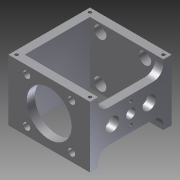
# Autodesk Inventor part: 13_0204_016
Saved by Autodesk Inventor 2012 SP1 (Build 160190100, 190)
## iProperties
Created: 2013-03-28
Part Number: 13_0204_016
Material: Default
Document SubType Name: Modeling
Designer: vogel
Density: 1 g/cm^3
Author: vogel
Autodesk Inventor part; units mm, degrees
note: some values were not read from the file. Chosen so that the rebuilt part matches the saved one: direction of "Bohrung2"; direction of "Bohrung3"; direction of "Bohrung4"; direction of "Bohrung5".
ref_plane "YZ Plane" through (0, 0, 0) normal (1, 0, 0) x (0, 1, 0)
ref_plane "XZ Plane" through (0, 0, 0) normal (0, 1, 0) x (-1, 0, 0)
sketch "Skizze1" plane through (0, 0, 0) normal (0, 0, 1) x (1, 0, 0)
  line L0 (-20, 20) -> (20, 20)
  line L1 (20, 20) -> (20, -20)
  line L2 (20, -20) -> (-20, -20)
  line L3 (-20, -20) -> (-20, 20)
  line L4 (-28, 0) -> (28, 0) projected
  line L5 (0, -28) -> (0, 28) projected
  line L6 (16, 16) -> (-16, 16)
  line L7 (-16, 16) -> (-16, -16)
  line L8 (-16, -16) -> (16, -16)
  line L9 (16, -16) -> (16, 16)
  point P0 (0, 0)
  dimension "d0" = 40
  dimension "d1" = 4
  constraints: 16 end point, 4 parallel, 3 perpendicular, 1 horizontal, 5 other
  measures "d0" distance of L2.end L0.start
  measures "d1" distance between parallel lines of L0 L6
extrude "Extrusion1" add sketch "Skizze1" along normal blind 30 contours L0 L5 L6 L7 L4 L3 | L0 L1 L4 L9 L6 L5 | L4 L7 L8 L5 L2 L3 | L1 L2 L5 L8 L9 L4
sketch "Skizze2" plane through (20, -20, 0) normal (1, 0, 0) x (0, 0, -1)
  line L0 (-30, 40) -> (-30, 0) projected
  line L1 (0, 0) -> (-30, 0) projected
  line L2 (0, 40) -> (-30, 40) projected
  line L3 (0, -8) -> (0, 48) projected
  line L4 (6, 20) -> (-36, 20) projected
  line L5 (-30, 36) -> (-28, 36)
  line L6 (-23, 31) -> (-23, 9)
  line L7 (-28, 4) -> (-30, 4)
  line L8 (-30, 4) -> (-30, 36)
  line L9 (0, 36) -> (-2, 36)
  line L10 (-7, 31) -> (-7, 9)
  line L11 (-2, 4) -> (0, 4)
  line L12 (0, 4) -> (0, 36)
  line L13 (-15, 40) -> (-15, 0)
  line L14 (0, 4) -> (-30, 4) projected
  arc A0 (-23, 31) -> (-28, 36) centre (-28, 31) ccw
  arc A1 (-28, 4) -> (-23, 9) centre (-28, 9) ccw
  arc A2 (-7, 9) -> (-2, 4) centre (-2, 9) ccw
  arc A3 (-2, 36) -> (-7, 31) centre (-2, 31) ccw
  point P0 (0, 20)
  dimension "d5" = 16
  dimension "d6" = 5
  constraints: 18 end point, 8 point on circle, 8 tangent, 4 centre point, 4 parallel, 3 collinear, 3 equal radius, 2 horizontal, 2 midpoint, 2 perpendicular, 2 point on line, 2 other
  measures "d5" distance between parallel lines of L10 L6
  measures "d6" radius of A0
extrude "Extrusion2" cut sketch "Skizze2" against normal up to surface (4 mm away) contours L5 A0 L6 L4 L0 | L4 L6 A1 L7 L0 | L3 L4 L10 A3 L9 | L4 L3 L11 A2 L10
sketch "Skizze4" plane through (20, -20, 0) normal (1, 0, 0) x (0, 0, -1)
  circle A0 centre (-20, 20) radius 1.15 projected
  circle A1 centre (-10, 20) radius 1.15 projected
  point P0 (0, 20)
  constraints: 2 coincident
hole "Bohrung2" at (20, 0, 20) at (20, 0, 10) direction (-1, 0, 0) diameter 1.567 end up to surface thread size "M2x0.4" class "6H" standard "ISO Metric profile"
sketch "Skizze5" plane through (20, -20, 0) normal (1, 0, 0) x (0, 0, -1)
  circle A0 centre (-15, 20) radius 2 projected
  point P0 (0, 20)
  constraints: 1 coincident
hole "Bohrung3" at (20, 0, 15) direction (-1, 0, 0) diameter 4.5 end up to surface
sketch "Skizze6" plane through (-20, -20, 0) normal (0, -1, 0) x (1, 0, 0)
  line L0 (40, 30) -> (0, 30) projected
  line L1 (0, 0) -> (0, 30) projected
  line L2 (40, 0) -> (40, 30) projected
  line L3 (40, 15) -> (0, 15)
  line L4 (20, 0) -> (20, 30)
  point P0 (20, 15)
  constraints: 4 end point, 4 midpoint
hole "Bohrung4" at (0, -20, 15) direction (0, 1, 0) diameter 22 end up to surface
sketch "Skizze7" plane through (20, -20, 0) normal (1, 0, 0) x (0, 0, -1)
  line L0 (0, 0) -> (-30, 0) projected
  line L1 (-7, 9) -> (-7, 31) projected
  line L2 (0, 40) -> (-30, 40) projected
  line L3 (-23, 31) -> (-23, 9) projected
  line L4 (-15, 0) -> (-15, 40)
  line L5 (-23, 20) -> (-7, 20)
  point P0 (0, 20)
  point P1 (-15, 11)
  point P2 (-15, 29)
  dimension "d43" = 18
  constraints: 4 end point, 4 midpoint, 2 point on line, 1 symmetric about line
  measures "d43" distance of point (-15, 29) point (-15, 11)
hole "Bohrung5" at (20, -9, 15) at (20, 9, 15) direction (-1, 0, 0) diameter 6.5 end up to surface
sketch "Skizze8" plane through (-20, -20, 0) normal (0, -1, 0) x (1, 0, 0)
  circle A0 centre (20, 15) radius 11 projected
  line L0 (9, 26) -> (31, 26)
  line L1 (31, 26) -> (31, 4)
  line L2 (31, 4) -> (9, 4)
  line L3 (9, 4) -> (9, 26)
  line L4 (-8, 0) -> (48, 0) projected
  line L5 (20, -6) -> (20, 36) projected
  line L6 (20, 15) -> (29.164, 15)
  point P0 (20, 0)
  dimension "d51" = 22
  constraints: 10 end point, 4 coincident, 3 perpendicular, 2 parallel, 1 horizontal, 2 other
  measures "d51" distance of L0.start L0.end
hole "Bohrung6" at (-11, -20, 26) at (11, -20, 26) at (11, -20, 4) at (-11, -20, 4) direction (0, 1, 0) diameter 3.4 end through all
sketch "Skizze9" plane through (-20, 20, 0) normal (0, 1, 0) x (1, 0, 0)
  circle A0 centre (9, -4) radius 1.7 projected
  circle A1 centre (31, -4) radius 1.7 projected
  circle A2 centre (31, -26) radius 1.7 projected
  circle A3 centre (9, -26) radius 1.7 projected
  point P0 (20, 0)
  constraints: 4 coincident
hole "Bohrung7" at (-11, 20, 4) at (11, 20, 4) at (11, 20, 26) at (-11, 20, 26) direction (0, -1, 0) diameter 6 depth 8 tip angle 118
sketch "Skizze10" plane through (0, 0, 30) normal (0, 0, 1) x (1, 0, 0)
  line L0 (20, 20) -> (20, 16) projected
  line L1 (-20, 20) -> (20, 20) projected
  line L2 (-20, -20) -> (-20, 20) projected
  line L3 (20, -20) -> (-20, -20) projected
  line L4 (-18, 18) -> (18, 18)
  line L5 (18, 18) -> (18, -18)
  line L6 (18, -18) -> (-18, -18)
  line L7 (-18, -18) -> (-18, 18)
  point P0 (0, 0)
  dimension "d66" = 2
  dimension "d67" = 2
  dimension "d68" = 2
  dimension "d69" = 2
  constraints: 8 end point, 4 coincident, 2 parallel, 1 horizontal, 1 perpendicular
  measures "d66" distance between parallel lines of L2 L7
  measures "d67" distance between parallel lines of L1 L4
  measures "d68" distance between parallel lines of L0 L5
  measures "d69" distance between parallel lines of L6 L3
hole "Bohrung8" at (-18, 18, 30) at (18, 18, 30) at (18, -18, 30) at (-18, -18, 30) direction (0, 0, -1) diameter 1.567 depth 8 tip angle 118 thread size "M2x0.4" class "6H" standard "ISO Metric profile"
ref_plane "Arbeitsebene1" through (0, 0, 15) normal (0, 0, 1) x (1, 0, 0)
mirror "Spiegeln1" about plane through (0, 0, 15) normal (0, 0, 1) of "Bohrung8"
